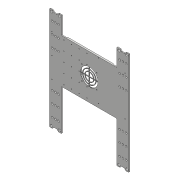
# Autodesk Inventor part: Chassis_Ceiling
Saved by Autodesk Inventor 2018 (Build 220112000, 112)
## iProperties
Created: 2019-09-19
Part Number: Chassis_Ceiling
Material: Generic
Document SubType Name: Modeling
Designer: Clevo
Density: 1 g/cm^3
Appearance: Default
Author: Clevo
Autodesk Inventor part; units mm, degrees
ref_plane "YZ Plane" through (0, 0, 0) normal (1, 0, 0) x (0, 1, 0)
ref_plane "XZ Plane" through (0, 0, 0) normal (0, 1, 0) x (-1, 0, 0)
ref_plane "XY Plane" through (0, 0, 0) normal (0, 0, 1) x (1, 0, 0)
sketch "Sketch1" plane through (0, 0, 0) normal (0, 1, 0) x (-1, 0, 0)
  line L0 (-86, -111.4) -> (86, -111.4)
  line L1 (86, -111.4) -> (86, 111.4)
  line L2 (86, 111.4) -> (-86, 111.4)
  line L3 (-86, 111.4) -> (-86, -111.4)
  line L4 (-86, -111.4) -> (86, 111.4) construction
  line L5 (86, -111.4) -> (-86, 111.4) construction
  point P0 (0, 0)
  dimension "d0" = 172
  dimension "d1" = 222.8
  constraints: 12 end point, 2 midpoint, 2 parallel, 1 horizontal, 1 perpendicular
  measures "d0" distance of L1.end L2.end
  measures "d1" distance of L0.end L1.end
extrude "Extrusion1" add sketch "Sketch1" along normal blind 2
sketch "Sketch2" plane through (0, 2, 0) normal (0, 1, 0) x (1, 0, 0)
  line L0 (64.5687, 107.3624) -> (82.0312, 107.3624)
  line L1 (82.0312, 107.3624) -> (82.0312, -107.3624)
  line L2 (82.0312, -107.3624) -> (64.5687, -107.3624)
  line L3 (64.5687, -107.3624) -> (64.5687, 107.3624)
  line L4 (64.5687, 107.3624) -> (82.0312, -107.3624) construction
  line L5 (82.0312, 107.3624) -> (64.5687, -107.3624) construction
  point P0 (0, 0)
  point P1 (73.3, 0)
  point P2 (73.3, 0)
  dimension "d4" = 214.7248
  dimension "d5" = 17.4625
  dimension "d6" = 64.5687
  constraints: 12 end point, 3 midpoint, 2 parallel, 1 horizontal, 1 horizontal alignment, 1 perpendicular
  measures "d4" distance of L0.end L1.end
  measures "d5" distance of L1.end L2.end
  measures "d6" distance from line of point (0, 0) L3
hole "Hole1" at (64.5687, 2, -107.3624) at (82.0312, 2, -107.3624) at (64.5687, 2, 107.3624) at (82.0312, 2, 107.3624) direction (0, -1, 0) diameter 5.3 depth 8 tip angle 118 clearance for "Flat Head Machine Screw" size "M5" standard "Ansi Metric M Profile"
mirror "Mirror1" about plane through (0, 0, 0) normal (1, 0, 0) of "Hole1"
sketch "Sketch3" plane through (0, 2, 0) normal (0, 1, 0) x (1, 0, 0)
  line L0 (86, 111.4) -> (-86, 111.4) projected
  line L1 (80, 111.4) -> (76.3938, 107.7938)
  line L2 (76.3938, 107.7938) -> (70.2938, 107.7938)
  line L3 (70.2938, 107.7938) -> (66.6875, 111.4)
  point P0 (0, 0)
  dimension "d14" = 5.1
  dimension "d15" = 5.1
  dimension "d16" = 6.1
  dimension "d17" = 6
  constraints: 6 end point, 2 point on line, 1 parallel, 1 perpendicular
  measures "d14" distance of L1.start L1.end
  measures "d15" distance of L2.end L3.end
  measures "d16" distance of L1.end L2.end
  measures "d17" distance of L0.start L1.start
extrude "Extrusion2" cut sketch "Sketch3" against normal through all
sketch "Sketch4" plane through (0, 2, 0) normal (0, 1, 0) x (1, 0, 0)
  line L0 (66.6875, 111.4) -> (-86, 111.4) projected
  line L1 (60, 111.4) -> (-60, 111.4)
  line L2 (-60, 111.4) -> (-60, 22.6)
  line L3 (-60, 22.6) -> (60, 22.6)
  line L4 (60, 22.6) -> (60, 111.4)
  point P0 (0, 0)
  point P1 (0, 22.6)
  dimension "d20" = 120
  dimension "d21" = 88.8
  constraints: 8 end point, 2 parallel, 1 horizontal, 1 midpoint, 1 perpendicular, 1 point on line, 1 vertical alignment
  measures "d20" distance of L2.end L3.end
  measures "d21" distance of L3.end L1.start
extrude "Extrusion3" cut sketch "Sketch4" against normal through all
mirror "Mirror2" about plane through (0, 0, 0) normal (1, 0, 0) of "Extrusion2"
sketch "Sketch11" plane through (0, 0, 0) normal (0, -1, 0) x (1, 0, 0)
  line L0 (-86, 111.4) -> (86, 111.4) projected
  line L1 (60, 73.4) -> (-60, 73.4)
  line L2 (-60, 73.4) -> (-60, 111.4)
  line L3 (-60, 111.4) -> (60, 111.4)
  line L4 (60, 111.4) -> (60, 73.4)
  line L5 (60, 73.4) -> (-60, 111.4) construction
  line L6 (-60, 73.4) -> (60, 111.4) construction
  point P0 (0, 0)
  point P1 (0, 92.4)
  point P2 (0, 92.4)
  dimension "d87" = 120
  dimension "d88" = 38
  constraints: 12 end point, 3 midpoint, 2 parallel, 1 horizontal, 1 perpendicular, 1 point on line, 1 vertical alignment
  measures "d87" distance of L1.start L1.end
  measures "d88" distance of L1.end L2.end
extrude "Extrusion6" cut sketch "Sketch11" against normal through all
fillet "Fillet1" radius 1 12 edges at (86, 1, 111.4) (86, 1, -111.4) (80, 1, -111.4) (66.6875, 1, -111.4) (60, 1, -111.4) (-60, 1, -111.4) (-66.6875, 1, -111.4) (-80, 1, -111.4) (-86, 1, -111.4) (-86, 1, 111.4) (-60, 1, 111.4) (60, 1, 111.4)
fillet "Fillet1" radius 1 8 edges at (60, 1, 73.4) (76.3938, 1, -107.7938) (-76.3938, 1, -107.7938) (-70.2938, 1, -107.7938) (-60, 1, -22.6) (60, 1, -22.6) (70.2938, 1, -107.7938) (-60, 1, 73.4)
sketch "Sketch5" plane through (0, 0, 0) normal (0, -1, 0) x (1, 0, 0)
  line L0 (73.3, -90.7) -> (73.3, -39.9)
  circle A0 centre (82.0312, -107.3624) radius 2.65 projected
  line L1 (86, 110.4) -> (86, -110.4) projected
  point P0 (0, 0)
  point P1 (73.3, -65.3)
  dimension "d26" = 50.8
  dimension "d28" = 12.7
  dimension "d94" = 42.0624
  constraints: 2 end point, 1 midpoint, 1 vertical
  measures "d26" distance of L0.start L0.end
  measures "d28" distance between parallel lines of L0 L1
  measures "d94" vertical distance of A0.centre point (73.3, -65.3)
hole "Hole2" at (73.3, 0, -65.3) at (73.3, 0, -90.7) at (73.3, 0, -39.9) direction (0, 1, 0) diameter 4.3 end through all clearance for "Flat Head Machine Screw" size "M4" standard "Ansi Metric M Profile"
pattern_linear "Rectangular Pattern1" count 2 spacing 7 along (1, 0, 0) count 2 spacing 7 along (-1, 0, 0) of "Hole2"
mirror "Mirror4" about plane through (0, 0, 0) normal (0, 0, 1) of "Hole2", "Rectangular Pattern1"
mirror "Mirror5" about plane through (0, 0, 0) normal (1, 0, 0) of "Hole2", "Rectangular Pattern1", "Mirror4"
sketch "Sketch6" plane through (0, 2, 0) normal (0, 1, 0) x (1, 0, 0)
  line L0 (59, -73.4) -> (-59, -73.4) projected
  line L1 (-50, 22.6) -> (50, 22.6)
  line L2 (50, 22.6) -> (50, -73.4)
  line L3 (50, -73.4) -> (-50, -73.4)
  line L4 (-50, -73.4) -> (-50, 22.6)
  line L5 (-50, 22.6) -> (50, -73.4) construction
  line L6 (50, 22.6) -> (-50, -73.4) construction
  line L7 (59, 22.6) -> (-59, 22.6) projected
  point P0 (0, 0)
  point P1 (0, -25.4)
  point P2 (0, -25.4)
  dimension "d91" = 100
  constraints: 12 end point, 3 midpoint, 2 parallel, 1 collinear, 1 horizontal, 1 perpendicular, 1 point on line, 1 vertical alignment
  measures "d91" distance between parallel lines of L4 L2
extrude "Extrusion4" add sketch "Sketch6" along normal blind 1.5
chamfer "Chamfer1" distance 1.5 angle 45 2 edges at (50, 2, 25.4) (-50, 2, 25.4)
fillet "Fillet2" radius 3 10 edges at (-51.4999, 2, 25.4) (-50, 3.5, -22.6) (-50, 3.4999, 73.4) (-50, 3.4999, 25.4) (-50, 3.5, 25.4) (51.4999, 2, 25.4) (50, 3.5, -22.6) (50, 3.5, 25.4) (50, 3.4999, 25.4) (50, 3.5, 73.4)
sketch "Sketch7" plane through (0, 0, 0) normal (0, -1, 0) x (1, 0, 0)
  circle A0 centre (-66.3, 90.7) radius 2.15 projected
  circle A1 centre (-66.3, 39.9) radius 2.15 projected
  circle A2 centre (-66.3, 65.3) radius 2.15 projected
  circle A3 centre (-80.3, 90.7) radius 2.15 projected
  circle A4 centre (-80.3, 39.9) radius 2.15 projected
  circle A5 centre (-80.3, 65.3) radius 2.15 projected
  circle A6 centre (-73.3, 90.7) radius 2.15 projected
  circle A7 centre (-73.3, 39.9) radius 2.15 projected
  circle A8 centre (-73.3, 65.3) radius 2.15 projected
  circle A9 centre (-66.3, -90.7) radius 2.15 projected
  circle A10 centre (-66.3, -39.9) radius 2.15 projected
  circle A11 centre (-66.3, -65.3) radius 2.15 projected
  circle A12 centre (-80.3, -90.7) radius 2.15 projected
  circle A13 centre (-80.3, -39.9) radius 2.15 projected
  circle A14 centre (-80.3, -65.3) radius 2.15 projected
  circle A15 centre (-73.3, -90.7) radius 2.15 projected
  circle A16 centre (-73.3, -39.9) radius 2.15 projected
  circle A17 centre (-73.3, -65.3) radius 2.15 projected
  circle A18 centre (66.3, 90.7) radius 2.15 projected
  circle A19 centre (66.3, 39.9) radius 2.15 projected
  circle A20 centre (66.3, 65.3) radius 2.15 projected
  circle A21 centre (80.3, 90.7) radius 2.15 projected
  circle A22 centre (80.3, 39.9) radius 2.15 projected
  circle A23 centre (80.3, 65.3) radius 2.15 projected
  circle A24 centre (73.3, 90.7) radius 2.15 projected
  circle A25 centre (73.3, 39.9) radius 2.15 projected
  circle A26 centre (73.3, 65.3) radius 2.15 projected
  circle A27 centre (66.3, -90.7) radius 2.15 projected
  circle A28 centre (66.3, -39.9) radius 2.15 projected
  circle A29 centre (66.3, -65.3) radius 2.15 projected
  circle A30 centre (80.3, -90.7) radius 2.15 projected
  circle A31 centre (80.3, -39.9) radius 2.15 projected
  circle A32 centre (73.3, -90.7) radius 2.15 projected
  circle A33 centre (73.3, -65.3) radius 2.15 projected
  circle A34 centre (73.3, -39.9) radius 2.15 projected
  line L0 (-85, 111.4) -> (-61, 111.4) projected
  line L1 (61, 111.4) -> (85, 111.4) projected
  arc A35 (-85, 111.4) -> (-86, 110.4) centre (-85, 110.4) ccw projected
  line L2 (-86, -110.4) -> (-86, 110.4) projected
  arc A36 (-86, -110.4) -> (-85, -111.4) centre (-85, -110.4) ccw projected
  line L3 (-80.4142, -111.4) -> (-85, -111.4) projected
  arc A37 (-80.4142, -111.4) -> (-79.7071, -111.1071) centre (-80.4142, -110.4) ccw projected
  line L4 (-79.7071, -111.1071) -> (-76.6866, -108.0866) projected
  arc A38 (-75.9795, -107.7938) -> (-76.6866, -108.0866) centre (-75.9795, -108.7938) ccw projected
  line L5 (-75.9795, -107.7938) -> (-70.708, -107.7938) projected
  arc A39 (-70.0009, -108.0866) -> (-70.708, -107.7938) centre (-70.708, -108.7938) ccw projected
  line L6 (-70.0009, -108.0866) -> (-66.9804, -111.1071) projected
  arc A40 (-66.9804, -111.1071) -> (-66.2733, -111.4) centre (-66.2733, -110.4) ccw projected
  line L7 (-61, -111.4) -> (-66.2733, -111.4) projected
  arc A41 (-61, -111.4) -> (-60, -110.4) centre (-61, -110.4) ccw projected
  line L8 (-60, -110.4) -> (-60, -23.6) projected
  arc A42 (-59, -22.6) -> (-60, -23.6) centre (-59, -23.6) ccw projected
  line L9 (-59, -22.6) -> (59, -22.6) projected
  arc A43 (60, -23.6) -> (59, -22.6) centre (59, -23.6) ccw projected
  line L10 (60, -23.6) -> (60, -110.4) projected
  arc A44 (60, -110.4) -> (61, -111.4) centre (61, -110.4) ccw projected
  line L11 (66.2733, -111.4) -> (61, -111.4) projected
  arc A45 (66.2733, -111.4) -> (66.9804, -111.1071) centre (66.2733, -110.4) ccw projected
  line L12 (66.9804, -111.1071) -> (70.0009, -108.0866) projected
  arc A46 (70.708, -107.7938) -> (70.0009, -108.0866) centre (70.708, -108.7938) ccw projected
  line L13 (70.708, -107.7938) -> (75.9795, -107.7938) projected
  arc A47 (76.6866, -108.0866) -> (75.9795, -107.7938) centre (75.9795, -108.7938) ccw projected
  line L14 (76.6866, -108.0866) -> (79.7071, -111.1071) projected
  arc A48 (79.7071, -111.1071) -> (80.4142, -111.4) centre (80.4142, -110.4) ccw projected
  line L15 (85, -111.4) -> (80.4142, -111.4) projected
  arc A49 (85, -111.4) -> (86, -110.4) centre (85, -110.4) ccw projected
  line L16 (86, 110.4) -> (86, -110.4) projected
  arc A50 (86, 110.4) -> (85, 111.4) centre (85, 110.4) ccw projected
  circle A51 centre (82.0312, 107.3624) radius 2.65 projected
  circle A52 centre (82.0312, -107.3624) radius 2.65 projected
  circle A53 centre (64.5687, -107.3624) radius 2.65 projected
  circle A54 centre (64.5687, 107.3624) radius 2.65 projected
  circle A55 centre (-82.0312, 107.3624) radius 2.65 projected
  circle A56 centre (-82.0312, -107.3624) radius 2.65 projected
  circle A57 centre (-64.5687, -107.3624) radius 2.65 projected
  circle A58 centre (-64.5687, 107.3624) radius 2.65 projected
  line L17 (78, -14.6) -> (20, -14.6)
  line L18 (20, -14.6) -> (20, 71.4)
  line L19 (20, 71.4) -> (78, 71.4)
  line L20 (78, 71.4) -> (78, -14.6)
  arc A59 (61, 111.4) -> (60, 110.4) centre (61, 110.4) ccw projected
  line L21 (60, 110.4) -> (60, 74.4) projected
  arc A60 (59, 73.4) -> (60, 74.4) centre (59, 74.4) ccw projected
  line L22 (59, 73.4) -> (-59, 73.4) projected
  arc A61 (-60, 74.4) -> (-59, 73.4) centre (-59, 74.4) ccw projected
  line L23 (-60, 74.4) -> (-60, 110.4) projected
  arc A62 (-60, 110.4) -> (-61, 111.4) centre (-61, 110.4) ccw projected
  point P0 (0, 0)
  point P1 (20, 28.4)
  dimension "d49" = 58
  dimension "d50" = 86
  dimension "d58" = 28.4
  dimension "d59" = 8
  constraints: 8 end point, 2 parallel, 1 horizontal, 1 midpoint, 1 perpendicular
  measures "d49" distance of L17.start L17.end
  measures "d50" distance of L17.end L18.end
  measures "d58" vertical distance of point (0, 0) point (20, 28.4)
  measures "d59" distance between parallel lines of L16 L20
hole "Hole3" at (78, 0, -14.6) at (20, 0, -14.6) at (20, 0, 71.4) at (78, 0, 71.4) direction (0, 1, 0) diameter 1.567 end through all thread size "M2x0.4" class "6H" standard "ANSI Metric M Profile"
sketch "Sketch9" plane through (0, 0, 0) normal (0, -1, 0) x (1, 0, 0)
  line L0 (-5, -16.6) -> (-55, -16.6)
  line L1 (-59, -22.6) -> (59, -22.6) projected
  point P0 (0, 0)
  point P1 (-21.6667, -16.6)
  point P2 (-38.3333, -16.6)
  dimension "d62" = 50
  dimension "d63" = 16.6667
  dimension "d64" = 16.6667
  dimension "d65" = 16.6667
  dimension "d66" = 6
  dimension "d77" = 5
  constraints: 2 end point, 2 point on line, 1 horizontal
  measures "d62" distance of L0.start L0.end
  measures "d63" distance of L0.start point (-21.667, -16.6)
  measures "d64" distance of point (-38.333, -16.6) point (-21.667, -16.6)
  measures "d65" distance of L0.end point (-38.333, -16.6)
  measures "d66" distance between parallel lines of L1 L0
  measures "d77" horizontal distance of point (0, 0) L0.start
hole "Hole4" at (-21.6667, 0, -16.6) at (-38.3333, 0, -16.6) at (-5, 0, -16.6) at (-55, 0, -16.6) direction (0, 1, 0) diameter 1.567 end through all thread size "M2x0.4" class "6H" standard "ANSI Metric M Profile"
pattern_linear "Rectangular Pattern2" count 5 spacing 21 along (0, 0, 1) of "Hole4"
sketch "Sketch10" plane through (0, 0, 0) normal (0, -1, 0) x (1, 0, 0)
  line L0 (-81, -19.6) -> (-81, 70.4)
  line L1 (-86, -110.4) -> (-86, 110.4) projected
  point P0 (0, 0)
  point P1 (-81, 25.4)
  dimension "d78" = 90
  dimension "d79" = 5
  dimension "d92" = 25.4
  constraints: 2 end point, 1 midpoint
  measures "d78" distance of L0.start L0.end
  measures "d79" distance between parallel lines of L1 L0
  measures "d92" vertical distance of point (0, 0) point (-81, 25.4)
hole "Hole5" at (-81, 0, -19.6) at (-81, 0, 25.4) at (-81, 0, 70.4) direction (0, 1, 0) diameter 1.567 end through all thread size "M2x0.4" class "6H" standard "ANSI Metric M Profile"
mirror "Mirror6" about plane through (0, 0, 0) normal (0, 0, 1) of "Extrusion2", "Mirror2"
fillet "Fillet3" radius 2 8 edges at (80, 1, 111.4) (76.3938, 1, 107.7938) (70.2938, 1, 107.7938) (66.6875, 1, 111.4) (-66.6875, 1, 111.4) (-70.2938, 1, 107.7938) (-76.3938, 1, 107.7938) (-80, 1, 111.4)
sketch "Sketch12" plane through (0, 3.5, 0) normal (0, 1, 0) x (1, 0, 0)
  circle A0 centre (-5, -67.4) radius 0.7835 projected
  circle A1 centre (-38.3333, -67.4) radius 0.7835 projected
  circle A2 centre (-21.6667, -67.4) radius 0.7835 projected
  circle A3 centre (-5, -46.4) radius 0.7835 projected
  circle A4 centre (-38.3333, -46.4) radius 0.7835 projected
  circle A5 centre (-21.6667, -46.4) radius 0.7835 projected
  circle A6 centre (-5, -25.4) radius 0.7835 projected
  circle A7 centre (-38.3333, -25.4) radius 0.7835 projected
  circle A8 centre (-21.6667, -25.4) radius 0.7835 projected
  circle A9 centre (-5, -4.4) radius 0.7835 projected
  circle A10 centre (-38.3333, -4.4) radius 0.7835 projected
  circle A11 centre (-21.6667, -4.4) radius 0.7835 projected
  circle A12 centre (-5, 16.6) radius 0.7835 projected
  circle A13 centre (-21.6667, 16.6) radius 0.7835 projected
  circle A14 centre (-38.3333, 16.6) radius 0.7835 projected
  circle A15 centre (20, -71.4) radius 0.7835 projected
  circle A16 centre (20, 14.6) radius 0.7835 projected
  line L0 (48.774, 22.6) -> (48.774, -73.4) projected
  line L1 (48.774, 22.6) -> (-48.774, 22.6) projected
  line L2 (-48.774, -73.4) -> (-48.774, 22.6) projected
  line L3 (-48.774, -73.4) -> (48.774, -73.4) projected
  line L4 (-16, -41.4) -> (16, -41.4)
  line L5 (16, -41.4) -> (16, -9.4)
  line L6 (16, -9.4) -> (-16, -9.4)
  line L7 (-16, -9.4) -> (-16, -41.4)
  line L8 (-16, -41.4) -> (16, -9.4) construction
  line L9 (16, -41.4) -> (-16, -9.4) construction
  point P0 (0, 0)
  point P1 (0, -25.4)
  point P2 (0, -25.4)
  point P3 (0, -25.4)
  point P4 (-48.774, -25.4)
  dimension "d95" = 32
  dimension "d96" = 32
  constraints: 12 end point, 5 midpoint, 2 parallel, 1 horizontal, 1 horizontal alignment, 1 perpendicular, 1 vertical alignment
  measures "d95" distance of L5.end L6.end
  measures "d96" distance of L4.end L5.end
hole "Hole6" at (-16, 3.5, 9.4) at (16, 3.5, 9.4) at (-16, 3.5, 41.4) at (16, 3.5, 41.4) direction (0, -1, 0) diameter 2.459 end through all thread size "M3x0.5" class "6H" standard "ANSI Metric M Profile"
sketch "Sketch13" plane through (0, 3.5, 0) normal (0, 1, 0) x (1, 0, 0)
  circle A0 centre (-16, -41.4) radius 1.2295 projected
  circle A1 centre (-16, -9.4) radius 1.2295 projected
  circle A2 centre (16, -9.4) radius 1.2295 projected
  circle A3 centre (16, -41.4) radius 1.2295 projected
  circle A4 centre (-5, -67.4) radius 0.7835 projected
  circle A5 centre (-38.3333, -67.4) radius 0.7835 projected
  circle A6 centre (-21.6667, -67.4) radius 0.7835 projected
  circle A7 centre (-5, -46.4) radius 0.7835 projected
  circle A8 centre (-38.3333, -46.4) radius 0.7835 projected
  circle A9 centre (-21.6667, -46.4) radius 0.7835 projected
  circle A10 centre (-5, -25.4) radius 0.7835 projected
  circle A11 centre (-38.3333, -25.4) radius 0.7835 projected
  circle A12 centre (-21.6667, -25.4) radius 0.7835 projected
  circle A13 centre (-5, -4.4) radius 0.7835 projected
  circle A14 centre (-38.3333, -4.4) radius 0.7835 projected
  circle A15 centre (-21.6667, -4.4) radius 0.7835 projected
  circle A16 centre (-5, 16.6) radius 0.7835 projected
  circle A17 centre (-21.6667, 16.6) radius 0.7835 projected
  circle A18 centre (-38.3333, 16.6) radius 0.7835 projected
  circle A19 centre (20, -71.4) radius 0.7835 projected
  circle A20 centre (20, 14.6) radius 0.7835 projected
  line L0 (48.774, 22.6) -> (48.774, -73.4) projected
  line L1 (48.774, 22.6) -> (-48.774, 22.6) projected
  line L2 (-48.774, -73.4) -> (-48.774, 22.6) projected
  line L3 (-48.774, -73.4) -> (48.774, -73.4) projected
  circle A21 centre (16, -41.4) radius 1.2295 projected
  line L4 (-16, -9.4) -> (16, -9.4)
  line L5 (16, -9.4) -> (16, -41.4)
  line L6 (16, -41.4) -> (-16, -41.4)
  line L7 (-16, -41.4) -> (-16, -9.4)
  line L8 (-20.25, -5.15) -> (20.25, -5.15)
  line L9 (20.25, -5.15) -> (20.25, -45.65)
  line L10 (20.25, -45.65) -> (-20.25, -45.65)
  line L11 (-20.25, -45.65) -> (-20.25, -5.15)
  point P0 (0, 0)
  point P1 (-20.25, -25.4)
  point P2 (16, -25.4)
  point P3 (0, -5.15)
  point P4 (0, -9.4)
  dimension "d104" = 40.5
  dimension "d105" = 40.5
  constraints: 16 end point, 4 midpoint, 4 parallel, 2 horizontal, 2 perpendicular, 1 horizontal alignment, 1 vertical alignment
  measures "d104" distance of L8.start L8.end
  measures "d105" distance of L8.end L9.end
extrude "Extrusion7" cut sketch "Sketch13" against normal blind 2 contours L6 L7 A0 | A0 L7 L6 | A0 L7 A1 L4 A2 L5 A3 L6 | L6 L5 A3 | A3 L5 L6 | L7 L4 A1 | A1 L4 L7 | L5 L4 A2 | A2 L4 L5 | L10 A7 | A7 L10 L11 L8 A13 L9 | A13 L8 | A10 picked at (-5.0255, -45.6401) picked at (-4.9745, -5.1599)
fillet "Fillet4" radius 1 4 edges at (-4.7733, 2.5, 5.15) (-5.2267, 2.5, 5.15) (-5.2267, 2.5, 45.65) (-4.7733, 2.5, 45.65)
fillet "Fillet5" radius 0.5 4 edges at (20.25, 2.5, 5.15) (-20.25, 2.5, 5.15) (-20.25, 2.5, 45.65) (20.25, 2.5, 45.65)
sketch "Sketch14" plane through (0, 1.5, 0) normal (0, 1, 0) x (1, 0, 0)
  arc A0 (19.75, -45.65) -> (20.25, -45.15) centre (19.75, -45.15) ccw projected
  line L0 (20.25, -5.65) -> (20.25, -45.15) projected
  arc A1 (20.25, -5.65) -> (19.75, -5.15) centre (19.75, -5.65) ccw projected
  line L1 (-3.2341, -5.15) -> (19.75, -5.15) projected
  arc A2 (-4.2242, -4.2902) -> (-3.2341, -5.15) centre (-3.2341, -4.15) ccw projected
  arc A3 (-5.7758, -4.2902) -> (-4.2242, -4.2902) centre (-5, -4.4) ccw projected
  arc A4 (-6.7659, -5.15) -> (-5.7758, -4.2902) centre (-6.7659, -4.15) ccw projected
  line L2 (-19.75, -5.15) -> (-6.7659, -5.15) projected
  arc A5 (-19.75, -5.15) -> (-20.25, -5.65) centre (-19.75, -5.65) ccw projected
  line L3 (-20.25, -45.15) -> (-20.25, -5.65) projected
  arc A6 (-20.25, -45.15) -> (-19.75, -45.65) centre (-19.75, -45.15) ccw projected
  line L4 (-6.7659, -45.65) -> (-19.75, -45.65) projected
  arc A7 (-5.7758, -46.5098) -> (-6.7659, -45.65) centre (-6.7659, -46.65) ccw projected
  arc A8 (-4.2242, -46.5098) -> (-5.7758, -46.5098) centre (-5, -46.4) ccw projected
  arc A9 (-3.2341, -45.65) -> (-4.2242, -46.5098) centre (-3.2341, -46.65) ccw projected
  line L5 (19.75, -45.65) -> (-3.2341, -45.65) projected
  circle A10 centre (-5, -25.4) radius 0.7835 projected
  circle A11 centre (16, -41.4) radius 1.2295 projected
  circle A12 centre (16, -9.4) radius 1.2295 projected
  circle A13 centre (-16, -9.4) radius 1.2295 projected
  circle A14 centre (-16, -41.4) radius 1.2295 projected
  circle A15 centre (0, -25.4) radius 19
  line L6 (-20.25, -45.15) -> (-20.25, -5.65) projected
  line L7 (48.774, 22.6) -> (-48.774, 22.6) projected
  point P0 (0, 0)
  point P1 (-20.25, -25.4)
  point P2 (0, 22.6)
  dimension "d110" = 38
  constraints: 2 midpoint, 1 centre point, 1 horizontal alignment, 1 vertical alignment
  measures "d110" diameter of A15
extrude "Extrusion8" cut sketch "Sketch14" against normal through all contours A15
fillet "Fillet6" radius 0.5 1 edges at (-19, 1.5, 25.4)
sketch "Sketch15" plane through (0, 0, 0) normal (0, -1, 0) x (1, 0, 0)
  circle A0 centre (0, 25.4) radius 19 projected
  circle A1 centre (-16, 41.4) radius 1.2295 projected
  circle A2 centre (-16, 9.4) radius 1.2295 projected
  circle A3 centre (16, 9.4) radius 1.2295 projected
  circle A4 centre (16, 41.4) radius 1.2295 projected
  arc A5 (-79.4142, 110.8142) -> (-80.8284, 111.4) centre (-80.8284, 109.4) ccw projected
  line L0 (-85, 111.4) -> (-80.8284, 111.4) projected
  arc A6 (-85, 111.4) -> (-86, 110.4) centre (-85, 110.4) ccw projected
  line L1 (-86, -110.4) -> (-86, 110.4) projected
  arc A7 (-86, -110.4) -> (-85, -111.4) centre (-85, -110.4) ccw projected
  line L2 (-80.4142, -111.4) -> (-85, -111.4) projected
  arc A8 (-80.4142, -111.4) -> (-79.7071, -111.1071) centre (-80.4142, -110.4) ccw projected
  line L3 (-79.7071, -111.1071) -> (-76.6866, -108.0866) projected
  arc A9 (-75.9795, -107.7938) -> (-76.6866, -108.0866) centre (-75.9795, -108.7938) ccw projected
  line L4 (-75.9795, -107.7938) -> (-70.708, -107.7938) projected
  arc A10 (-70.0009, -108.0866) -> (-70.708, -107.7938) centre (-70.708, -108.7938) ccw projected
  line L5 (-70.0009, -108.0866) -> (-66.9804, -111.1071) projected
  arc A11 (-66.9804, -111.1071) -> (-66.2733, -111.4) centre (-66.2733, -110.4) ccw projected
  line L6 (-61, -111.4) -> (-66.2733, -111.4) projected
  arc A12 (-61, -111.4) -> (-60, -110.4) centre (-61, -110.4) ccw projected
  line L7 (-60, -110.4) -> (-60, -23.6) projected
  arc A13 (-59, -22.6) -> (-60, -23.6) centre (-59, -23.6) ccw projected
  line L8 (-59, -22.6) -> (59, -22.6) projected
  arc A14 (60, -23.6) -> (59, -22.6) centre (59, -23.6) ccw projected
  line L9 (60, -23.6) -> (60, -110.4) projected
  arc A15 (60, -110.4) -> (61, -111.4) centre (61, -110.4) ccw projected
  line L10 (66.2733, -111.4) -> (61, -111.4) projected
  arc A16 (66.2733, -111.4) -> (66.9804, -111.1071) centre (66.2733, -110.4) ccw projected
  line L11 (66.9804, -111.1071) -> (70.0009, -108.0866) projected
  arc A17 (70.708, -107.7938) -> (70.0009, -108.0866) centre (70.708, -108.7938) ccw projected
  line L12 (70.708, -107.7938) -> (75.9795, -107.7938) projected
  arc A18 (76.6866, -108.0866) -> (75.9795, -107.7938) centre (75.9795, -108.7938) ccw projected
  line L13 (76.6866, -108.0866) -> (79.7071, -111.1071) projected
  arc A19 (79.7071, -111.1071) -> (80.4142, -111.4) centre (80.4142, -110.4) ccw projected
  line L14 (85, -111.4) -> (80.4142, -111.4) projected
  arc A20 (85, -111.4) -> (86, -110.4) centre (85, -110.4) ccw projected
  line L15 (86, 110.4) -> (86, -110.4) projected
  arc A21 (86, 110.4) -> (85, 111.4) centre (85, 110.4) ccw projected
  line L16 (80.8284, 111.4) -> (85, 111.4) projected
  arc A22 (80.8284, 111.4) -> (79.4142, 110.8142) centre (80.8284, 109.4) ccw projected
  line L17 (79.4142, 110.8142) -> (76.9795, 108.3795) projected
  arc A23 (75.5653, 107.7938) -> (76.9795, 108.3795) centre (75.5653, 109.7938) ccw projected
  line L18 (75.5653, 107.7938) -> (71.1222, 107.7938) projected
  arc A24 (69.708, 108.3795) -> (71.1222, 107.7938) centre (71.1222, 109.7938) ccw projected
  line L19 (69.708, 108.3795) -> (67.2733, 110.8142) projected
  arc A25 (67.2733, 110.8142) -> (65.8591, 111.4) centre (65.8591, 109.4) ccw projected
  line L20 (61, 111.4) -> (65.8591, 111.4) projected
  arc A26 (61, 111.4) -> (60, 110.4) centre (61, 110.4) ccw projected
  line L21 (60, 110.4) -> (60, 74.4) projected
  arc A27 (59, 73.4) -> (60, 74.4) centre (59, 74.4) ccw projected
  line L22 (59, 73.4) -> (-59, 73.4) projected
  arc A28 (-60, 74.4) -> (-59, 73.4) centre (-59, 74.4) ccw projected
  line L23 (-60, 74.4) -> (-60, 110.4) projected
  arc A29 (-60, 110.4) -> (-61, 111.4) centre (-61, 110.4) ccw projected
  line L24 (-65.8591, 111.4) -> (-61, 111.4) projected
  arc A30 (-65.8591, 111.4) -> (-67.2733, 110.8142) centre (-65.8591, 109.4) ccw projected
  line L25 (-67.2733, 110.8142) -> (-69.708, 108.3795) projected
  arc A31 (-71.1222, 107.7938) -> (-69.708, 108.3795) centre (-71.1222, 109.7938) ccw projected
  line L26 (-71.1222, 107.7938) -> (-75.5653, 107.7938) projected
  arc A32 (-76.9795, 108.3795) -> (-75.5653, 107.7938) centre (-75.5653, 109.7938) ccw projected
  line L27 (-76.9795, 108.3795) -> (-79.4142, 110.8142) projected
  circle A33 centre (-81, 25.4) radius 0.7835 projected
  circle A34 centre (-81, -19.6) radius 0.7835 projected
  circle A35 centre (-81, 70.4) radius 0.7835 projected
  circle A36 centre (-5, 67.4) radius 0.7835 projected
  circle A37 centre (-55, 67.4) radius 0.7835 projected
  circle A38 centre (-38.3333, 67.4) radius 0.7835 projected
  circle A39 centre (-21.6667, 67.4) radius 0.7835 projected
  circle A40 centre (-5, 46.4) radius 0.7835 projected
  circle A41 centre (-55, 46.4) radius 0.7835 projected
  circle A42 centre (-38.3333, 46.4) radius 0.7835 projected
  circle A43 centre (-21.6667, 46.4) radius 0.7835 projected
  circle A44 centre (-55, 25.4) radius 0.7835 projected
  circle A45 centre (-38.3333, 25.4) radius 0.7835 projected
  circle A46 centre (-21.6667, 25.4) radius 0.7835 projected
  circle A47 centre (-5, 4.4) radius 0.7835 projected
  circle A48 centre (-55, 4.4) radius 0.7835 projected
  circle A49 centre (-38.3333, 4.4) radius 0.7835 projected
  circle A50 centre (-21.6667, 4.4) radius 0.7835 projected
  circle A51 centre (-5, -16.6) radius 0.7835 projected
  circle A52 centre (-21.6667, -16.6) radius 0.7835 projected
  circle A53 centre (-38.3333, -16.6) radius 0.7835 projected
  circle A54 centre (-55, -16.6) radius 0.7835 projected
  circle A55 centre (20, 71.4) radius 0.7835 projected
  circle A56 centre (78, -14.6) radius 0.7835 projected
  circle A57 centre (20, -14.6) radius 0.7835 projected
  circle A58 centre (78, 71.4) radius 0.7835 projected
  circle A59 centre (-66.3, 90.7) radius 2.15 projected
  circle A60 centre (-66.3, 39.9) radius 2.15 projected
  circle A61 centre (-66.3, 65.3) radius 2.15 projected
  circle A62 centre (-80.3, 90.7) radius 2.15 projected
  circle A63 centre (-80.3, 39.9) radius 2.15 projected
  circle A64 centre (-80.3, 65.3) radius 2.15 projected
  circle A65 centre (-73.3, 90.7) radius 2.15 projected
  circle A66 centre (-73.3, 39.9) radius 2.15 projected
  circle A67 centre (-73.3, 65.3) radius 2.15 projected
  circle A68 centre (-66.3, -90.7) radius 2.15 projected
  circle A69 centre (-66.3, -39.9) radius 2.15 projected
  circle A70 centre (-66.3, -65.3) radius 2.15 projected
  circle A71 centre (-80.3, -90.7) radius 2.15 projected
  circle A72 centre (-80.3, -39.9) radius 2.15 projected
  circle A73 centre (-80.3, -65.3) radius 2.15 projected
  circle A74 centre (-73.3, -90.7) radius 2.15 projected
  circle A75 centre (-73.3, -39.9) radius 2.15 projected
  circle A76 centre (-73.3, -65.3) radius 2.15 projected
  circle A77 centre (66.3, 90.7) radius 2.15 projected
  circle A78 centre (66.3, 39.9) radius 2.15 projected
  circle A79 centre (66.3, 65.3) radius 2.15 projected
  circle A80 centre (80.3, 90.7) radius 2.15 projected
  circle A81 centre (80.3, 39.9) radius 2.15 projected
  circle A82 centre (80.3, 65.3) radius 2.15 projected
  circle A83 centre (73.3, 90.7) radius 2.15 projected
  circle A84 centre (73.3, 39.9) radius 2.15 projected
  circle A85 centre (73.3, 65.3) radius 2.15 projected
  circle A86 centre (66.3, -90.7) radius 2.15 projected
  circle A87 centre (66.3, -39.9) radius 2.15 projected
  circle A88 centre (66.3, -65.3) radius 2.15 projected
  circle A89 centre (80.3, -90.7) radius 2.15 projected
  circle A90 centre (80.3, -39.9) radius 2.15 projected
  circle A91 centre (80.3, -65.3) radius 2.15 projected
  circle A92 centre (73.3, -90.7) radius 2.15 projected
  circle A93 centre (73.3, -65.3) radius 2.15 projected
  circle A94 centre (73.3, -39.9) radius 2.15 projected
  circle A95 centre (-64.5687, 107.3624) radius 2.65 projected
  circle A96 centre (-64.5687, -107.3624) radius 2.65 projected
  circle A97 centre (-82.0312, -107.3624) radius 2.65 projected
  circle A98 centre (-82.0312, 107.3624) radius 2.65 projected
  circle A99 centre (64.5687, 107.3624) radius 2.65 projected
  circle A100 centre (64.5687, -107.3624) radius 2.65 projected
  circle A101 centre (82.0312, -107.3624) radius 2.65 projected
  circle A102 centre (82.0312, 107.3624) radius 2.65 projected
  line L28 (0.5, 5.4) -> (-0.5, 5.4)
  line L29 (-0.5, 5.4) -> (-0.5, 45.4)
  line L30 (-0.5, 45.4) -> (0.5, 45.4)
  line L31 (0.5, 45.4) -> (0.5, 5.4)
  line L32 (0.5, 5.4) -> (-0.5, 45.4) construction
  line L33 (-0.5, 5.4) -> (0.5, 45.4) construction
  line L34 (-20, 24.9) -> (20, 24.9)
  line L35 (20, 24.9) -> (20, 25.9)
  line L36 (20, 25.9) -> (-20, 25.9)
  line L37 (-20, 25.9) -> (-20, 24.9)
  line L38 (-20, 24.9) -> (20, 25.9) construction
  line L39 (20, 24.9) -> (-20, 25.9) construction
  circle A103 centre (0, 25.4) radius 10
  circle A104 centre (0, 25.4) radius 9
  circle A105 centre (0, 25.4) radius 15
  circle A106 centre (0, 25.4) radius 14
  point P0 (0, 0)
  dimension "d114" = 1
  dimension "d115" = 40
  dimension "d116" = 40
  dimension "d117" = 1
  dimension "d118" = 20
  dimension "d119" = 18
  dimension "d120" = 28
  dimension "d121" = 30
  constraints: 24 end point, 4 centre point, 4 coincident, 4 midpoint, 4 parallel, 2 horizontal, 2 perpendicular
  measures "d114" distance of L29.end L30.end
  measures "d115" distance of L30.end L28.start
  measures "d116" distance of L35.end L36.end
  measures "d117" distance of L34.end L35.end
  measures "d118" diameter of A103
  measures "d119" diameter of A104
  measures "d120" diameter of A106
  measures "d121" diameter of A105
extrude "Extrusion9" add sketch "Sketch15" against normal blind 1 contours A0 L34 A105 L36 | A0 L36 L35 L34 | L31 A105 L29 A0 | A0 L29 L30 L31 | A105 L34 A106 L36 | L36 A106 L31 A105 | L31 L28 L29 A0 | A0 L29 A105 L31 | A105 L31 A106 L34 | L31 A106 L29 A105 | A106 L34 A103 L36 | A105 L29 A106 L31 | L36 A105 L34 A0 | A0 L34 L37 L36 | L29 A106 L36 A105 | L31 A103 L29 A106 | A103 L34 A104 L36 | L36 A104 L31 A103 | A105 L34 A106 L29 | A106 L29 A103 L31 | A103 L31 A104 L34 | L36 A106 L34 A105 | L31 A104 L29 A103 | A104 L34 L31 L36 | A103 L29 A104 L31 | L36 A103 L34 A106 | L29 A104 L36 A103 | L31 L36 L29 A104 | L31 L34 L29 L36 | A103 L34 A104 L29 | A104 L29 L34 L31 | L36 A104 L34 A103 | L29 L34 A104 L36
equation "\"d15\" = d14"
equation "\"d63\" = d65"
equation "\"d64\" = d63"
equation "\"d96\" = d95"
equation "\"d105\" = d104"
body "Solid1"
